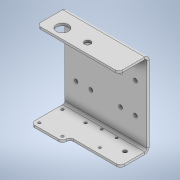
# Autodesk Inventor part: arm_bracket
Saved by Autodesk Inventor 2020 (Build 240168000, 168)
## iProperties
Created: 2020-08-30
Part Number: arm_bracket
Material: Generic
Document SubType Name: Sheet Metal
Designer: s4393944
Density: 1 g/cm^3
Sheet Metal Rule: Default_mm
Appearance: Default
Author: s4393944
Autodesk Inventor part; units mm, degrees
ref_plane "YZ Plane" through (0, 0, 0) normal (1, 0, 0) x (0, 1, 0)
ref_plane "XZ Plane" through (0, 0, 0) normal (0, 1, 0) x (-1, 0, 0)
ref_plane "XY Plane" through (0, 0, 0) normal (0, 0, 1) x (1, 0, 0)
sketch "Sketch2" plane through (0, 0, 0) normal (0, 0, 1) x (1, 0, 0)
  line L0 (0, 92) -> (-55, 92)
  line L1 (-55, 92) -> (-55, -100)
  line L2 (-55, -100) -> (-12.7, -100)
  line L3 (55, -90) -> (55, 92)
  line L4 (55, 92) -> (0, 92)
  line L5 (-12.7, -100) -> (-12.7, -90)
  line L6 (-12.7, -90) -> (55, -90)
  point P0 (0, 0)
  dimension "d4" = 55
  dimension "d5" = 55
  dimension "d6" = 92
  dimension "d7" = 192
  dimension "d73" = 42.3
  dimension "d74" = 10
  measures "d4" horizontal distance of point (0, 0) L3.end
  measures "d5" horizontal distance of L0.end point (0, 0)
  measures "d6" vertical distance of L0.end point (0, 0)
  measures "d7" distance of L1.end L0.end
  measures "d73" distance between parallel lines of L1 L5
  measures "d74" distance of L2.end L5.end
extrude "Plate1" add sketch "Sketch2" along normal blind 3
sketch "Sketch4" plane through (0, 0, 3) normal (0, 0, 1) x (1, 0, 0)
  line L0 (55, -90) -> (55, 92) projected
  line L1 (55, 54) -> (-55, 54)
  line L2 (-55, 92) -> (-55, -100) projected
  point P0 (0, 0)
  dimension "d17" = 54
  constraints: 2 end point, 2 point on line, 1 horizontal
  measures "d17" vertical distance of point (0, 0) L1.start
fold "Fold2" angle 90 bend radius 3 thickness 3 k factor 0.44 line from (55, 54, 3) to (-55, 54, 3) line at bend centre moving side (0, 1, 0) folds toward (0, 0, 1)
sketch "Sketch5" plane through (0, 0, 3) normal (0, 0, 1) x (1, 0, 0)
  line L0 (-55, -100) -> (-55, 50.6071) projected
  line L1 (-55, -54) -> (55, -54)
  line L2 (55, -90) -> (55, 50.6071) projected
  point P0 (0, 0)
  dimension "d24" = 54
  constraints: 2 end point, 2 point on line, 1 horizontal
  measures "d24" vertical distance of L1.end point (0, 0)
fold "Fold3" angle 90 bend radius 3 thickness 3 k factor 0.44 line from (-55, -54, 3) to (55, -54, 3) line at bend centre moving side (0, -1, 0) folds toward (0, 0, 1)
sketch "Sketch6" plane through (0, 0, 3) normal (0, 0, 1) x (1, 0, 0)
  circle A0 centre (-19.85, 20.32) radius 2.55
  circle A1 centre (-19.85, -20.32) radius 2.55
  circle A2 centre (-39.85, 20.32) radius 2.55
  circle A3 centre (-39.85, -20.32) radius 2.55
  circle A4 centre (19.85, 20.32) radius 2.55
  circle A5 centre (39.85, 20.32) radius 2.55
  circle A6 centre (19.85, -20.32) radius 2.55
  circle A7 centre (39.85, -20.32) radius 2.55
  circle A8 centre (0, 0) radius 2.55
  dimension "d31" = 20.32
  dimension "d32" = 20.32
  dimension "d33" = 5.1
  dimension "d35" = 19.85
  dimension "d44" = 19.85
  dimension "d45" = 5.1
  dimension "d46" = 5.1
  dimension "d47" = 39.85
  dimension "d48" = 39.85
  dimension "d49" = 5.1
  dimension "d50" = 5.1
  dimension "d51" = 5.1
  dimension "d52" = 5.1
  dimension "d53" = 19.85
  dimension "d54" = 39.85
  dimension "d55" = 39.85
  dimension "d56" = 19.85
  dimension "d57" = 5.1
  constraints: 9 centre point, 1 coincident
  measures "d31" vertical distance of point (0, 0) A0.centre
  measures "d32" vertical distance of point (0, 0) A1.centre
  measures "d33" diameter of A0
  measures "d35" horizontal distance of point (0, 0) A0.centre
  measures "d44" horizontal distance of point (0, 0) A1.centre
  measures "d45" diameter of A2
  measures "d46" diameter of A3
  measures "d47" horizontal distance of point (0, 0) A2.centre
  measures "d48" horizontal distance of A3.centre point (0, 0)
  measures "d49" diameter of A4
  measures "d50" diameter of A5
  measures "d51" diameter of A6
  measures "d52" diameter of A7
  measures "d53" horizontal distance of point (0, 0) A4.centre
  measures "d54" horizontal distance of point (0, 0) A5.centre
  measures "d55" horizontal distance of point (0, 0) A7.centre
  measures "d56" horizontal distance of point (0, 0) A6.centre
  measures "d57" diameter of A8
hole "Hole1" at (-19.85, 20.32, 3) at (-19.85, -20.32, 3) at (-39.85, 20.32, 3) at (-39.85, -20.32, 3) at (19.85, 20.32, 3) at (39.85, 20.32, 3) at (19.85, -20.32, 3) at (39.85, -20.32, 3) direction (0, 0, -1) diameter 5.1 end through all
sketch "Sketch7" plane through (-55, 56.6071, 40.6071) normal (0, 1, 0) x (1, 0, 0)
  circle A0 centre (21.15, 13.15) radius 8.1
  line L0 (0, 0) -> (0, 34.6071) projected
  line L1 (110, 0) -> (0, 0) projected
  circle A1 centre (55, 13.15) radius 4.25
  line L2 (110, 34.6071) -> (0, 34.6071) projected
  line L3 (42.3, 2) -> (42.3, -8) projected
  line L4 (0, -8) -> (0, 34.6071) projected
  line L5 (42.3, -8) -> (0, -8) projected
  point P0 (55, 40.6071)
  point P1 (0, 37.6071)
  dimension "d61" = 8.5
  dimension "d62" = 0
  dimension "d135" = 33.85
  dimension "d154" = 21.15
  constraints: 2 centre point, 1 other
  measures "d61" diameter of A1
  measures "d62" horizontal distance of point (55, 40.607) A1.centre
  measures "d135" distance of A1.centre A0.centre
  measures "d154" distance from line of L5 A1.centre
hole "Hole2" at (0, 56.6071, 27.4571) direction (0, -1, 0) diameter 8.2 depth 3 tip angle 118
fillet "Corner Round1" radius 5 6 edges at (-55, -55.1071, 48.6071) (-12.7, -55.1071, 48.6071) (55, -55.1071, 38.6071) (55, 55.1071, 40.6071) (-55, 55.1071, 40.6071) (-12.7, -55.1071, 38.6071)
sketch "Sketch9" plane through (-55, -56.6071, 6) normal (0, -1, 0) x (1, 0, 0)
  circle A0 centre (55, 2.6071) radius 1.55
  circle A1 centre (75, 25.1071) radius 1.55
  circle A2 centre (75, 2.6071) radius 1.55
  line L0 (47.3, 32.6071) -> (105, 32.6071) projected
  line L1 (5, 42.6071) -> (37.3, 42.6071) projected
  line L2 (110, 27.6071) -> (110, 0) projected
  line L3 (110, -6) -> (0, -6) projected
  point P0 (55, -6)
  dimension "d104" = 3.1
  dimension "d105" = 3.1
  dimension "d106" = 3.1
  dimension "d107" = 30
  dimension "d108" = 40
  dimension "d109" = 7.5
  dimension "d110" = 30
  dimension "d111" = 35
  dimension "d112" = 35
  dimension "d123" = 55
  constraints: 3 centre point
  measures "d104" diameter of A1
  measures "d105" diameter of A2
  measures "d106" diameter of A0
  measures "d107" distance from line of L0 A0.centre
  measures "d108" distance from line of L1 A0.centre
  measures "d109" distance from line of L0 A1.centre
  measures "d110" distance from line of L0 A2.centre
  measures "d111" distance from line of L2 A1.centre
  measures "d112" distance from line of L2 A2.centre
  measures "d123" distance from line of L2 point (55, -6)
hole "Hole4" at (0, -56.6071, 8.6071) at (20, -56.6071, 31.1071) at (20, -56.6071, 8.6071) direction (0, 1, 0) diameter 3.1 depth 3 tip angle 118
sketch "Sketch10" plane through (-55, -56.6071, 6) normal (0, -1, 0) x (1, 0, 0)
  circle A0 centre (96.25, 12.6071) radius 2.55
  line L0 (110, 27.6071) -> (110, 0) projected
  line L1 (47.3, 32.6071) -> (105, 32.6071) projected
  point P0 (55, -6)
  dimension "d125" = 5.1
  dimension "d126" = 13.75
  dimension "d127" = 20
  constraints: 1 centre point
  measures "d125" diameter of A0
  measures "d126" distance from line of L0 A0.centre
  measures "d127" distance from line of L1 A0.centre
hole "Hole5" at (41.25, -56.6071, 18.6071) direction (0, 1, 0) diameter 5.1 depth 3 tip angle 118
sketch "Sketch11" plane through (-55, 56.6071, 6) normal (0, 1, 0) x (1, 0, 0)
  circle A0 centre (21.15, -21.4571) radius 8.1
  line L0 (0, -29.6071) -> (0, 0) projected
  line L1 (105, -34.6071) -> (5, -34.6071) projected
  line L2 (37.3, -42.6071) -> (5, -42.6071) projected
  point P0 (55, 6)
  dimension "d148" = 16.2
  dimension "d149" = 21.15
  dimension "d155" = 21.15
  constraints: 1 centre point
  measures "d148" diameter of A0
  measures "d149" distance from line of L0 A0.centre
  measures "d155" distance from line of L2 A0.centre
hole "Hole6" at (-33.85, 56.6071, 27.4571) direction (0, -1, 0) diameter 16.2 depth 3 tip angle 118
sketch "Sketch12" plane through (-55, -56.6071, 6) normal (0, -1, 0) x (1, 0, 0)
  circle A0 centre (5.65, 36.9571) radius 2.1
  circle A1 centre (36.65, 36.9571) radius 2.1
  circle A2 centre (5.7214, 5.9571) radius 2.1
  circle A3 centre (36.7214, 5.9571) radius 2.1
  line L0 (0, 0) -> (0, 37.6071) projected
  line L1 (5, 42.6071) -> (37.3, 42.6071) projected
  point P0 (55, -6)
  dimension "d164" = 4.2
  dimension "d165" = 4.2
  dimension "d166" = 4.2
  dimension "d167" = 4.2
  dimension "d168" = 5.65
  dimension "d169" = 31
  dimension "d170" = 31
  dimension "d171" = 31
  dimension "d172" = 31
  dimension "d173" = 5.65
  dimension "d174" = 5.65
  constraints: 4 centre point
  measures "d164" diameter of A0
  measures "d165" diameter of A1
  measures "d166" diameter of A2
  measures "d167" diameter of A3
  measures "d168" distance from line of A0.centre L0
  measures "d169" distance of A1.centre A0.centre
  measures "d170" vertical distance of A2.centre A0.centre
  measures "d171" vertical distance of A1.centre A3.centre
  measures "d172" distance of A2.centre A3.centre
  measures "d173" distance from line of L1 A0.centre
  measures "d174" distance from line of L1 A1.centre
hole "Hole7" at (-49.35, -56.6071, 42.9571) at (-18.35, -56.6071, 42.9571) at (-49.2786, -56.6071, 11.9571) at (-18.2786, -56.6071, 11.9571) direction (0, 1, 0) diameter 3.5 depth 3 tip angle 118
equation "\"d8\" = Thickness"
equation "\"d18\" = BendReliefWidth"
equation "\"d19\" = BendReliefDepth"
equation "\"d20\" = MinimumRemnant"
equation "\"d21\" = TransitionRadius"
equation "\"d23\" = BendRadius"
equation "\"d25\" = BendReliefWidth"
equation "\"d26\" = BendReliefDepth"
equation "\"d27\" = MinimumRemnant"
equation "\"d28\" = TransitionRadius"
equation "\"d30\" = BendRadius"
equation "\"d42\" = Thickness"
equation "\"d68\" = Thickness"
equation "\"d118\" = Thickness"
equation "\"d133\" = Thickness"
equation "\"d161\" = Thickness"
equation "\"d180\" = Thickness"
equation "\"BendRadius\" = Thickness"
equation "\"BendReliefWidth\" = Thickness"
equation "\"BendReliefDepth\" = 0.5 * Thickness"
equation "\"CornerReliefSize\" = 4 * Thickness"
equation "\"MinimumRemnant\" = 2 * Thickness"
equation "\"TransitionRadius\" = BendRadius"
equation "\"JacobiRadiusSize\" = BendRadius"
equation "\"GapSize\" = Thickness"
equation "\"Thickness\" = 3"
body "Solid1"
